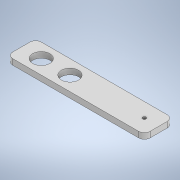
# Autodesk Inventor part: stationary arm
Saved by Autodesk Inventor 2022 (Build 260153000, 153)
## iProperties
Created: 2022-06-14
Part Number: stationary arm
Material: Generic
Document SubType Name: Modeling
Designer: chait
Density: 1 g/cm^3
Appearance: Default
Author: chait
Autodesk Inventor part; units mm, degrees
ref_plane "YZ Plane" through (0, 0, 0) normal (1, 0, 0) x (0, 1, 0)
ref_plane "XZ Plane" through (0, 0, 0) normal (0, 1, 0) x (-1, 0, 0)
ref_plane "XY Plane" through (0, 0, 0) normal (0, 0, 1) x (1, 0, 0)
sketch "Sketch1" plane through (0, 0, 0) normal (0, 1, 0) x (-1, 0, 0)
  line L0 (6, -1.25) -> (-6, -1.25)
  line L1 (-6, -1.25) -> (-6, 1.25)
  line L2 (-6, 1.25) -> (6, 1.25)
  line L3 (6, 1.25) -> (6, -1.25)
  line L4 (6, -1.25) -> (-6, 1.25) construction
  line L5 (-6, -1.25) -> (6, 1.25) construction
  point P0 (0, 0)
  dimension "d0" = 12
  dimension "d1" = 2.5
  constraints: 12 end point, 2 midpoint, 2 parallel, 1 horizontal, 1 perpendicular
  measures "d0" distance of L1.end L2.end
  measures "d1" distance of L0.end L1.end
extrude "Extrusion1" add sketch "Sketch1" along normal blind 0.5
sketch "Sketch2" plane through (0, 0.5, 0) normal (0, 1, 0) x (1, 0, 0)
  circle A0 centre (-4.2565, 0) radius 0.75
  point P0 (0, 0)
  dimension "d4" = 1.5
  constraints: 1 centre point
  measures "d4" diameter of A0
extrude "Extrusion2" cut sketch "Sketch2" against normal blind 0.5
sketch "Sketch3" plane through (0, 0.5, 0) normal (0, 1, 0) x (1, 0, 0)
  circle A0 centre (-1.7501, 0) radius 0.75
  circle A1 centre (4.2419, 0) radius 0.75
  circle A2 centre (1.7477, 0) radius 0.75
  point P0 (0, 0)
  dimension "d7" = 1.5
  dimension "d8" = 1.5
  dimension "d9" = 1.5
  constraints: 3 centre point
  measures "d7" diameter of A0
  measures "d8" diameter of A1
  measures "d9" diameter of A2
extrude "Extrusion3" cut sketch "Sketch3" against normal blind 0.5 contours A0
sketch "Sketch7" plane through (0, 0.5, 0) normal (0, 1, 0) x (1, 0, 0)
  circle A0 centre (4.7487, 0) radius 0.15
  point P0 (0, 0)
  dimension "d21" = 0.3
  constraints: 1 centre point
  measures "d21" diameter of A0
extrude "Extrusion7" cut sketch "Sketch7" against normal blind 2
fillet "Fillet2" radius 0.5 1 edges at (6, 0.25, 1.25)
fillet "Fillet3" radius 0.5 1 edges at (6, 0.25, -1.25)
fillet "Fillet4" radius 0.5 1 edges at (-6, 0.25, 1.25)
fillet "Fillet5" radius 0.5 1 edges at (-6, 0.25, -1.25)
body "Solid1"
